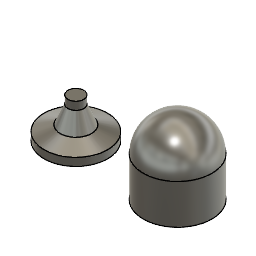
Learning revovle tool (Autodesk Fusion 360 design; units mm, degrees)
part number: 2025-11-30-21-15-05-836
Autodesk Fusion 360 part; units mm, degrees
sketch "Sketch1" plane through (0, 0, 0) normal (0, 0, 1) x (1, 0, 0)
  line L0 (0, 0) -> (0, 100)
  line L1 (0, 100) -> (20, 100)
  line L2 (20, 100) -> (20, 80)
  line L3 (20, 80) -> (39.1815, 34.8527)
  line L4 (39.1815, 34.8527) -> (80, 20)
  line L5 (80, 20) -> (80, 0)
  line L6 (80, 0) -> (0, 0)
  dimension "d1" = 100
  dimension "d2" = 20
  dimension "d3" = 133.014
  dimension "d4" = 49.0531
  dimension "d5" = 20
  dimension "d6" = 39.1815
  dimension "d7" = 20
  dimension "d8" = 80
  constraint coincident L0.start L6.end
  constraint vertical L0
  constraint perpendicular L0 L1
  constraint perpendicular L1 L2
  constraint parallel L2 L5
  constraint perpendicular L0 L6
  measures "d1" distance of L0.start L0.end
  measures "d2" distance of L0.end L1.end
  measures "d3" angle of L3 L4
  measures "d4" distance of L2.end L3.end
  measures "d5" distance of L4.end L5.end
  measures "d6" distance of L0 L3.end
  measures "d7" distance of L0 L2.end
  measures "d8" distance of L0 L4.end
revolve "Revolve1" add sketch "Sketch1" angle 360 about axis through (0, 0, 0) along (0, 1, 0) makes body 1
sketch "Sketch2" plane through (0, 0, 0) normal (0, 0, 1) x (1, 0, 0)
  line L0 (170, 0) -> (342.8773, 0)
  line L1 (342.8773, 0) -> (342.8773, 100)
  line L2 (342.8773, 100) -> (170, 100) construction
  line L3 (170, 100) -> (170, 0)
  arc A0 (342.8773, 100) -> (170, 100) centre (256.4386, 100) ccw
  line L4 (256.4386, 0) -> (256.4386, 186.4386)
  dimension "d10" = 100
  constraint horizontal L0
  constraint vertical L1
  constraint horizontal L2
  constraint vertical L3
  constraint tangent L3 A0
  constraint midpoint L0 L4.start
  constraint midpoint A0 L4.end
  measures "d10" distance of L0.start L2.end
revolve "Revolve2" add sketch "Sketch2" angle 360 about axis through (256.4386, 0, 0) along (0, 1, 0) separate body contours L0 L1 A0 L4 makes body 2
